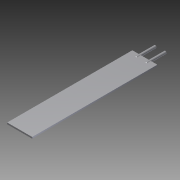
# Autodesk Inventor part: Ruler
Saved by Autodesk Inventor 2012 (Build 160160000, 160)
## iProperties
Created: 2013-07-07
Part Number: Ruler
Material: Default
Document SubType Name: Modeling
Designer: 1
Density: 1 g/cm^3
Author: 1
Autodesk Inventor part; units mm, degrees
ref_plane "YZ Plane" through (0, 0, 0) normal (1, 0, 0) x (0, 1, 0)
ref_plane "XZ Plane" through (0, 0, 0) normal (0, 1, 0) x (-1, 0, 0)
ref_plane "XY Plane" through (0, 0, 0) normal (0, 0, 1) x (1, 0, 0)
sketch "Sketch1" plane through (0, 0, 0) normal (0, 0, 1) x (1, 0, 0)
  arc A0 (12.5, 21.1789) -> (7.5, 21.1789) centre (10, 21.1789) ccw projected
  arc A1 (7.5, 21.1789) -> (12.5, 21.1789) centre (10, 21.1789) ccw projected
  arc A2 (-12.5, 21.1789) -> (-7.5, 21.1789) centre (-10, 21.1789) ccw projected
  arc A3 (-7.5, 21.1789) -> (-12.5, 21.1789) centre (-10, 21.1789) ccw projected
  line L0 (20, 16.9697) -> (20, 21.1789) projected
  line L1 (20, 25.3881) -> (20, 21.1789) projected
  line L2 (-20, 25.3881) -> (-20, 21.1789) projected
  line L3 (-20, 16.9697) -> (-20, 21.1789) projected
  line L4 (25, 19.6789) -> (-25, 19.6789)
  line L5 (-25, 19.6789) -> (-25, 22.6789)
  line L6 (-25, 22.6789) -> (25, 22.6789)
  line L7 (25, 22.6789) -> (25, 19.6789)
  line L8 (25, 22.6789) -> (-25, 19.6789) construction
  line L9 (-25, 22.6789) -> (25, 19.6789) construction
  line L10 (-20, 21.1789) -> (20, 21.1789) construction
  point P0 (0, 0)
  point P1 (0, 21.1789)
  dimension "d0" = 50
  dimension "d1" = 3
  constraints: 14 end point, 2 midpoint, 2 parallel, 2 perpendicular, 1 horizontal
  measures "d0" distance of L4.start L4.end
  measures "d1" distance of L6.end L4.start
extrude "Extrusion1" add sketch "Sketch1" along normal blind 250 contours A1 L4 A0 L6 | A0 L6 L1 L0 L4 A1 | A0 A1 L4 A2 A3 L6 | L6 L7 L4 L0 L1 | A3 A2 L4 L6 | A3 A2 L4 L3 L2 L6 | L2 L3 L4 L5 L6
sketch "Sketch2" plane through (0, 0, 0) normal (0, 0, -1) x (-1, 0, 0)
  arc A0 (-7.5, 21.1789) -> (-12.5, 21.1789) centre (-10, 21.1789) ccw projected
  arc A1 (-12.5, 21.1789) -> (-7.5, 21.1789) centre (-10, 21.1789) ccw projected
  arc A2 (12.5, 21.1789) -> (7.5, 21.1789) centre (10, 21.1789) ccw projected
  arc A3 (7.5, 21.1789) -> (12.5, 21.1789) centre (10, 21.1789) ccw projected
  circle A4 centre (-10, 21.1789) radius 2.5
  circle A5 centre (10, 21.1789) radius 2.5
  point P0 (0, 0)
  constraints: 2 coincident, 2 horizontal alignment, 4 other
extrude "Extrusion2" add sketch "Sketch2" along normal blind 30.925 and the other way blind 7.5255
fillet "Fillet1" radius 0.9 6 edges at (10, 22.6789, 7.5255) (8, 22.6789, 3.7628) (-8, 22.6789, 3.7628) (-10, 22.6789, 7.5255) (-12, 22.6789, 3.7628) (12, 22.6789, 3.7628)
fillet "Fillet2" radius 0.9 10 edges at (-12.0632, 22.7477, 8.0804) (-10, 23.6789, 7.5255) (-8.6948, 23.3111, 7.5663) (-7.9368, 22.7477, 8.0804) (-11.3052, 23.3112, 7.5662) (7.9368, 22.7477, 8.0804) (10, 23.6789, 7.5255) (11.3052, 23.3111, 7.5663) (12.0632, 22.7477, 8.0804) (8.6948, 23.3112, 7.5662)
body "Solid1"
